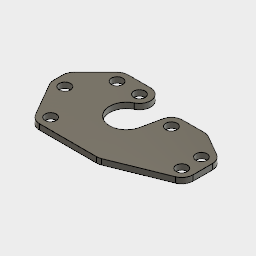
Tier 2 Practice Ex 3_ CSA011070∩╗┐ (Autodesk Fusion 360 design; units mm, degrees)
Autodesk Fusion 360 part; units mm, degrees
sketch "Sketch1" plane through (0, 0, 0) normal (0, 1, 0) x (1, 0, 0)
  line L0 (-101.6, 0) -> (-101.6, 19.0663)
  line L1 (-101.6, 19.0663) -> (-69.8663, 50.8)
  line L2 (-69.8663, 50.8) -> (-39.2395, 50.8)
  arc A0 (-33.7037, 26.67) -> (-39.2395, 50.8) centre (-39.2395, 38.1) ccw
  arc A1 (-33.7037, 26.67) -> (-6.7663, 5.5643) centre (-25.4, 9.525) ccw
  line L3 (-6.7663, 5.5643) -> (0, 37.3972)
  line L4 (0, 37.3972) -> (38.1, 37.3972)
  line L5 (38.1, 37.3972) -> (69.85, 19.0663)
  line L6 (69.85, 19.0663) -> (69.85, -19.05)
  line L7 (69.85, -19.05) -> (0, -47.2712)
  line L8 (0, -47.2712) -> (-74.3079, -47.2712)
  line L9 (-74.3079, -47.2712) -> (-101.6, 0)
  dimension "d1" = 9.525
  dimension "d2" = 19.05
  dimension "d3" = 25.4
  dimension "d4" = 102
  dimension "d5" = 38.1
  dimension "d6" = 150
  dimension "d7" = 69.85
  dimension "d8" = 112
  dimension "d9" = 19.05
  dimension "d10" = 120
  dimension "d11" = 101.6
  dimension "d12" = 135
  dimension "d13" = 50.8
  dimension "d14" = 12.7
  measures "d1" distance of origin A1.centre
  measures "d2" radius of A1
  measures "d3" distance of origin A1.centre
  measures "d4" angle of L3 L4
  measures "d5" distance of L3.end L4.end
  measures "d6" angle of L4 L5
  measures "d7" distance of origin L6
  measures "d8" angle of L6 L7
  measures "d9" distance of origin L6.end
  measures "d10" angle of L8 L9
  measures "d11" distance of origin L0
  measures "d12" angle of L0 L1
  measures "d13" distance of origin L2
  measures "d14" radius of A0
extrude "Extrude1" add sketch "Sketch1" along normal blind 6.35
fillet "Fillet1" radius 12.7 9 edges at (-69.8663, 3.175, -50.8) (-101.6, 3.175, -19.0663) (-101.6, 3.175, 0) (-74.3079, 3.175, 47.2712) (0, 3.175, 47.2712) (0, 3.175, -37.3972) (38.1, 3.175, -37.3972) (69.85, 3.175, -19.0663) (69.85, 3.175, 19.05)
sketch "Sketch2" plane through (0, 6.35, 0) normal (0, 1, 0) x (-1, 0, 0)
  arc A0 (-61.9075, 22.259) -> (-69.85, 10.4837) centre (-57.15, 10.4837) ccw
  line L0 (-69.85, 10.4837) -> (-69.85, -11.7339)
  arc A1 (-69.85, -11.7339) -> (-63.5, -22.7325) centre (-57.15, -11.7339) ccw
  line L1 (-63.5, -22.7325) -> (-41.047, -35.6957)
  arc A2 (-41.047, -35.6957) -> (-34.697, -37.3972) centre (-34.697, -24.6972) ccw
  line L2 (-34.697, -37.3972) -> (-10.2843, -37.3972)
  arc A3 (-10.2843, -37.3972) -> (2.1382, -27.3376) centre (-10.2843, -24.6972) ccw
  line L3 (2.1382, -27.3376) -> (6.7663, -5.5643)
  arc A4 (33.7037, -26.67) -> (6.7663, -5.5643) centre (25.4, -9.525) ccw
  arc A5 (33.7037, -26.67) -> (39.2395, -50.8) centre (39.2395, -38.1) ccw
  line L4 (39.2395, -50.8) -> (64.6058, -50.8)
  arc A6 (64.6058, -50.8) -> (73.586, -47.0803) centre (64.6058, -38.1) ccw
  line L5 (73.586, -47.0803) -> (97.8803, -22.786)
  arc A7 (97.8803, -22.786) -> (101.6, -13.8058) centre (88.9, -13.8058) ccw
  line L6 (101.6, -13.8058) -> (101.6, -3.403)
  arc A8 (101.6, -3.403) -> (99.8985, 2.947) centre (88.9, -3.403) ccw
  line L7 (99.8985, 2.947) -> (77.9741, 40.9212)
  arc A9 (77.9741, 40.9212) -> (66.9756, 47.2712) centre (66.9756, 34.5712) ccw
  line L8 (66.9756, 47.2712) -> (2.4686, 47.2712)
  arc A10 (2.4686, 47.2712) -> (-2.2889, 46.3465) centre (2.4686, 34.5712) ccw
  line L9 (-2.2889, 46.3465) -> (-61.9075, 22.259)
  circle A11 centre (64.6058, -38.1) radius 6.35
  circle A12 centre (39.2395, -38.1) radius 6.35
  circle A13 centre (-10.2843, -24.6972) radius 6.35
  circle A14 centre (-57.15, -11.7339) radius 6.35
  circle A15 centre (-57.15, 10.4837) radius 6.35
  circle A16 centre (66.9756, 34.5712) radius 6.35
  circle A17 centre (88.9, -3.403) radius 6.35
  dimension "d18" = 12.7
  measures "d18" diameter of A15
extrude "Extrude2" cut sketch "Sketch2" against normal blind 15.24 contours A11 | A12 | A13 | A14 | A15 | A16 | A17
